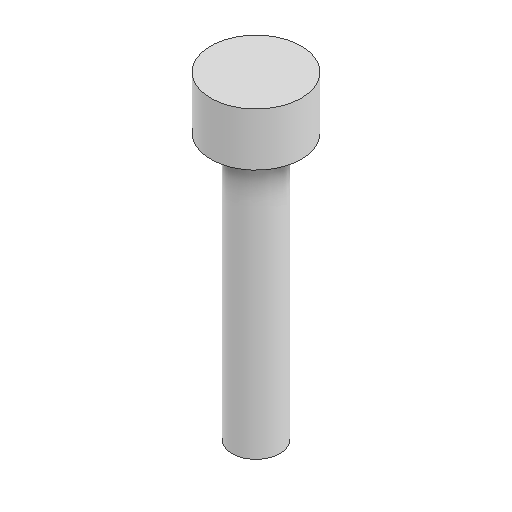
# Autodesk Inventor part: Screw 2
Saved by Autodesk Inventor 2025 (Build 290162010, 162A)
## iProperties
Created: 2024-12-04
Part Number: Screw 2
Material: Generic
Document SubType Name: Modeling
Designer: ALEXANDERNICHOLS
Density: 1 g/cm^3
Appearance: Default
Author: ALEXANDERNICHOLS
Autodesk Inventor part; units mm, degrees
ref_plane "YZ Plane" through (0, 0, 0) normal (1, 0, 0) x (0, 1, 0)
ref_plane "XZ Plane" through (0, 0, 0) normal (0, 1, 0) x (-1, 0, 0)
ref_plane "XY Plane" through (0, 0, 0) normal (0, 0, 1) x (1, 0, 0)
sketch "Sketch1" plane through (0, 0, 0) normal (0, 0, 1) x (1, 0, 0)
  line L0 (0, 0) -> (1.778, 0)
  line L1 (1.778, 0) -> (1.778, 19.7612)
  line L2 (1.778, 19.7612) -> (3.3655, 19.7612)
  line L3 (3.3655, 19.7612) -> (3.3655, 23.6982)
  line L4 (3.3655, 23.6982) -> (0, 23.6982)
  line L5 (0, 23.6982) -> (0, 0)
  dimension "d1" = 6.731
  dimension "d2" = 3.556
  dimension "d3" = 3.937
  dimension "d4" = 19.7612
  constraints: 12 end point, 4 perpendicular, 1 horizontal, 1 vertical
  measures "d1" diameter of L3 L5
  measures "d2" diameter of L1 L5
  measures "d3" distance of L2.end L3.end
  measures "d4" distance of L0.end L1.end
revolve "Revolution1" add sketch "Sketch1" angle 360 about axis through (0, 23.6982, 0) along (0, -1, 0)
body "Solid1"
